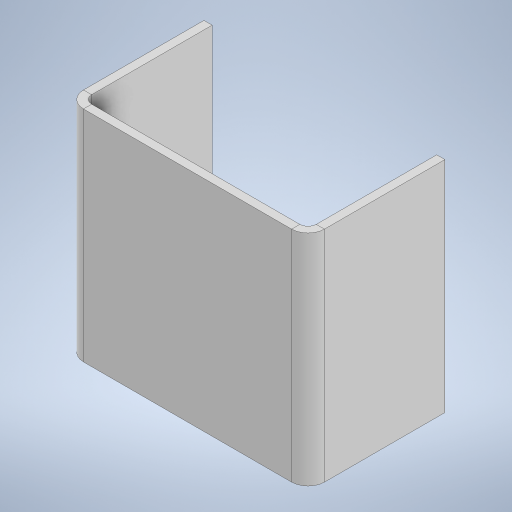
# Autodesk Inventor part: chest_cover_board_top
Saved by Autodesk Inventor 2024.1 (Build 281209000, 209)
## iProperties
Created: 2024-02-15
Part Number: chest_cover_board_top
Material: 一般
Document SubType Name: Sheet Metal
Designer: hibik
Density: 1 g/cm^3
Sheet Metal Rule: Default
Appearance: 既定
Author: hibik
Autodesk Inventor part; units mm, degrees
ref_plane "YZ Plane" through (0, 0, 0) normal (1, 0, 0) x (0, 1, 0)
ref_plane "XZ Plane" through (0, 0, 0) normal (0, 1, 0) x (-1, 0, 0)
ref_plane "XY Plane" through (0, 0, 0) normal (0, 0, 1) x (1, 0, 0)
sketch "スケッチ1" plane through (0, 0, 0) normal (0, 0, 1) x (1, 0, 0)
  line L0 (-22, 20) -> (22, 20)
  line L1 (22, 20) -> (22, -20)
  line L2 (22, -20) -> (-22, -20)
  line L3 (-22, -20) -> (-22, 20)
  line L4 (-22, 20) -> (22, -20) construction
  line L5 (22, 20) -> (-22, -20) construction
  point P0 (0, 0)
  point P1 (0, 0)
  dimension "d0" = 44
  dimension "d1" = 40
  measures "d0" distance of L1.end L2.end
  measures "d1" distance of L0.end L1.end
extrude "プレート1" add sketch "スケッチ1" along normal blind 1.5
sketch "スケッチ2" plane through (20.5, -20, 1.5) normal (1, 0, 0) x (0, 1, 0)
  line L0 (40, 0) -> (0, 0)
  line L1 (0, 0) -> (0, -25)
  line L2 (0, -25) -> (40, -25)
  line L3 (40, -25) -> (40, 0)
  constraints: 6 end point, 1 horizontal, 1 perpendicular, 1 vertical
edge flange "フランジ1" height 25 angle 90 thickness 1.5 bend radius 1.5 thickness toward (1, 0, 0) relief tear relief width 1.5 relief depth 0.75 corner gap 1.5 corner form 0 edges at (22, 0, 0) (-22, 0, 0) wall of the first edge with corners at (20.5, 20, 1.5) (20.5, -20, 1.5) (20.5, -20, -23.5) (20.5, 20, -23.5)
bend "曲げ1"
corner "コーナー1"
equation "\"BendRadius\" = Thickness"
equation "\"BendReliefWidth\" = Thickness"
equation "\"BendReliefDepth\" = 0.5 * Thickness"
equation "\"CornerReliefSize\" = 4 * Thickness"
equation "\"MinimumRemnant\" = 2 * Thickness"
equation "\"TransitionRadius\" = BendRadius"
equation "\"JacobiRadiusSize\" = BendRadius"
equation "\"GapSize\" = Thickness"
